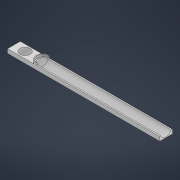
# Autodesk Inventor part: Trilho 60 minutos  - 12 horas
Saved by Autodesk Inventor 2022 (Build 260153000, 153)
## iProperties
Created: 2023-05-09
Part Number: Trilho 60 minutos  - 12 horas
Material: Genérico
Document SubType Name: Modeling
Designer: jpjoa
Density: 1 g/cm^3
Appearance: Padrão
Author: jpjoa
Autodesk Inventor part; units mm, degrees
ref_plane "YZ Plane" through (0, 0, 0) normal (1, 0, 0) x (0, 1, 0)
ref_plane "XZ Plane" through (0, 0, 0) normal (0, 1, 0) x (-1, 0, 0)
ref_plane "XY Plane" through (0, 0, 0) normal (0, 0, 1) x (1, 0, 0)
sketch "Esboço2" plane through (0, 0, 0) normal (0, 1, 0) x (-1, 0, 0)
  line L0 (-42.3088, 0) -> (-245.4, 0)
  line L1 (-245.4, 0) -> (-245.4, -20.4)
  line L2 (-245.4, -20.4) -> (-42.3088, -20.4)
  line L3 (-47.4, -19.2) -> (-245.4, -19.2)
  line L4 (-245.4, -1.2) -> (-47.4, -1.2)
  circle A0 centre (-47.4, -10.2) radius 9
  line L5 (-56.4, -20.4) -> (-56.4, -19.2)
  line L6 (-56.4, -1.2) -> (-56.4, 0)
  arc A1 (-42.3088, -20.4) -> (-42.3088, 0) centre (-47.4, -10.2) ccw
  arc A2 (-47.4, -20.4) -> (-47.4, 0) centre (-47.4, -10.2) ccw
  line L7 (-42.3088, 0) -> (0, 0)
  line L8 (0, 0) -> (0, -20.4)
  line L9 (0, -20.4) -> (-42.3088, -20.4)
  circle A3 centre (-18, -10.2) radius 9
  point P0 (0, -10.2)
  point P1 (-42.3088, -20.4)
  dimension "d6" = 20.4
  dimension "d8" = 1.2
  dimension "d11" = 1.2
  dimension "d25" = 18
  dimension "d44" = 1.2
  dimension "d45" = 1.2
  dimension "d46" = 198
  dimension "d47" = 36
  dimension "d48" = 18
  dimension "d49" = 18
  constraints: 20 end point, 8 point on line, 6 point on circle, 5 perpendicular, 4 centre point, 3 tangent, 2 horizontal, 2 horizontal alignment, 2 vertical, 1 coincident, 1 midpoint
  measures "d6" distance of L0.end L1.end
  measures "d8" distance between parallel lines of L2 L3
  measures "d11" distance between parallel lines of L0 L4
  measures "d25" diameter of A0
  measures "d44" radial gap between concentric circles of A2 A1
  measures "d45" radial gap between concentric circles of A0 A2
  measures "d46" distance from line of L1 A0.centre
  measures "d47" distance edge to line of A1 L8
  measures "d48" diameter of A3
  measures "d49" distance from line of L8 A3.centre
extrude "Extrusão1" add sketch "Esboço2" against normal blind 1.2 contours A1 L2 A2 L0 | L7 L8 L9 A1 | A2 L2 L5 L3 A0 L4 L6 L0 | L6 L4 L1 L0 | L4 A0 L3 L1 | L2 L1 L3 L5 | A0 | A3
extrude "Extrusão2" add sketch "Esboço2" along normal blind 9 contours L7 L8 L9 A1 | A2 L2 L5 L3 A0 L4 L6 L0 | L6 L4 L1 L0 | L2 L1 L3 L5
fillet "Arredondamento6" radius 9 4 edges at (146.4, 0, -1.2) (146.4, 0, -19.2) (38.4, 0, -10.2) (27, 0, -10.2)
sketch "Esboço6" plane through (0, -1.2, 0) normal (0, 0, 1) x (1, 0, 0)
  line L0 (245.4, 10.2) -> (0, 10.2)
  line L1 (0, 10.2) -> (0, 6.6)
  line L2 (0, 6.6) -> (245.4, 6.6)
  line L3 (245.4, 6.6) -> (245.4, 10.2)
  line L4 (245.4, 1.2) -> (245.4, 10.2) projected
  line L5 (0, 10.2) -> (0, 0) projected
  line L6 (47.4, 10.2) -> (245.4, 10.2) projected
  line L7 (47.4, 1.2) -> (245.4, 1.2) projected
  point P0 (0, 1.2)
  point P1 (245.4, 8.4)
  point P2 (245.4, 5.7)
  point P3 (0, 8.4)
  point P4 (0, 5.1)
  point P5 (122.7, 10.2)
  point P6 (146.4, 10.2)
  dimension "d50" = 5.4
  constraints: 8 end point, 6 midpoint, 2 perpendicular, 2 vertical alignment, 1 horizontal, 1 horizontal alignment, 1 vertical
  measures "d50" distance between parallel lines of L7 L2
extrude "Extrusão8" cut sketch "Esboço6" against normal up to surface (20.4 mm away)
extrude "Extrusão9" add sketch "Esboço2" along normal blind 9 contours A1 L2 A2 L0
equation "\"d6\" = Diâmetro_esfera + 2 * Margem"
equation "\"d8\" = Margem"
equation "\"d11\" = Margem"
equation "\"d25\" = Diâmetro_esfera"
equation "\"d44\" = Margem"
equation "\"d45\" = Margem"
equation "\"d46\" = 11 * Diâmetro_esfera"
equation "\"d47\" = 2 * Diâmetro_esfera"
equation "\"d48\" = Diâmetro_esfera"
equation "\"d49\" = 0.5 * d47"
equation "\"d13\" = Margem"
equation "\"d15\" = 0.5 * Diâmetro_esfera"
equation "\"d55\" = 0.5 * Diâmetro_esfera"
equation "\"d50\" = 0.3 * Diâmetro_esfera"
equation "\"d53\" = 0.5 * Diâmetro_esfera"
equation "\"Diâmetro_esfera\" = 18"
equation "\"Margem\" = 3 * Filamento"
equation "\"Filamento\" = 0.4"
equation "\"Parafuso\" = 3"
equation "\"d42\" = Margem"
equation "\"d43\" = Margem"
